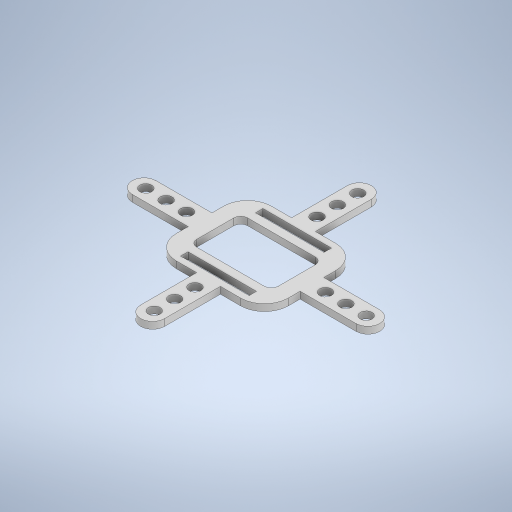
# Autodesk Inventor part: SoporteMarkers12
Saved by Autodesk Inventor 2024.3 (Build 283343000, 343)
## iProperties
Created: 2024-07-19
Part Number: SoporteMarkers12
Material: Generic
Document SubType Name: Modeling
Designer: pjcaa
Density: 1 g/cm^3
Appearance: Default
Mass: 1.30972 g
Surface Area: 17.5643 cm^2
Volume: 1.30972 cm^3
Author: pjcaa
Autodesk Inventor part; units mm, degrees
ref_plane "YZ Plane" through (0, 0, 0) normal (1, 0, 0) x (0, 1, 0)
ref_plane "XZ Plane" through (0, 0, 0) normal (0, 1, 0) x (-1, 0, 0)
ref_plane "XY Plane" through (0, 0, 0) normal (0, 0, 1) x (1, 0, 0)
sketch "Sketch1" plane through (0, 0, 0) normal (0, 1, 0) x (-1, 0, 0)
  line L0 (0, 0) -> (33, 0)
  line L1 (33, 0) -> (33, -28)
  line L2 (33, -28) -> (0, -28)
  line L3 (0, -28) -> (0, 0)
  line L4 (0, -17.5) -> (-20, -17.5)
  line L5 (-20, -17.5) -> (-20, -10.5)
  line L6 (-20, -10.5) -> (0, -10.5)
  line L7 (0, -10.5) -> (0, -17.5)
  line L8 (33, -17.5) -> (53, -17.5)
  line L9 (53, -17.5) -> (53, -10.5)
  line L10 (53, -10.5) -> (33, -10.5)
  line L11 (33, -10.5) -> (33, -17.5)
  line L12 (20, -28) -> (13, -28)
  line L13 (13, -28) -> (13, -48)
  line L14 (13, -48) -> (20, -48)
  line L15 (20, -48) -> (20, -28)
  line L16 (20, 0) -> (13, 0)
  line L17 (13, 0) -> (13, 20)
  line L18 (13, 20) -> (20, 20)
  line L19 (20, 20) -> (20, 0)
  circle A0 centre (16.5, -44) radius 1.75
  circle A1 centre (-16, -14) radius 1.75
  circle A2 centre (16.5, 16) radius 1.75
  circle A3 centre (49, -14) radius 1.75
  line L20 (16.5, -44) -> (16.5, -48) construction
  line L21 (-16, -14) -> (-20, -14) construction
  line L22 (16.5, 16) -> (16.5, 20) construction
  line L23 (49, -14) -> (53, -14) construction
  circle A4 centre (43, -14) radius 1.75
  circle A5 centre (37, -14) radius 1.75
  circle A6 centre (16.5, -38) radius 1.75
  circle A7 centre (16.5, -32) radius 1.75
  circle A8 centre (-10, -14) radius 1.75
  circle A9 centre (-4, -14) radius 1.75
  circle A10 centre (16.5, 10) radius 1.75
  circle A11 centre (16.5, 4) radius 1.75
  point P0 (16.5, -28)
  point P1 (16.5, 0)
  point P2 (0, -14)
  point P3 (33, -14)
  dimension "d0" = 33
  dimension "d1" = 28
  dimension "d29" = 7
  dimension "d34" = 20
  dimension "d35" = 4
  dimension "d36" = 3.5
  dimension "d44" = 6
  dimension "d51" = 6
  dimension "d58" = 6
  dimension "d65" = 6
  constraints: 48 end point, 14 perpendicular, 12 centre point, 12 midpoint, 10 parallel, 7 horizontal, 3 equal radius, 3 vertical alignment, 2 horizontal alignment, 2 vertical, 16 other
  measures "d0" distance of L1.end L2.end
  measures "d1" distance of L0.end L1.end
  measures "d29" distance of L8.end L9.end
  measures "d34" distance of L9.end L10.end
  measures "d35" distance of L20.start L20.end
  measures "d36" diameter of A0
  measures "d44" distance of L23.start A4.centre
  measures "d51" distance of L20.start A6.centre
  measures "d58" distance of L21.start A8.centre
  measures "d65" distance of L22.start A10.centre
extrude "Extrusion1" add sketch "Sketch1" along normal blind 2
sketch "Sketch2" plane through (0, 2, 0) normal (0, 1, 0) x (1, 0, 0)
  line L0 (0, 28) -> (-13, 28) projected
  line L1 (-33, 28) -> (-33, 17.5) projected
  line L2 (-33, 0) -> (-20, 0) projected
  line L3 (0, 0) -> (0, 10.5) projected
  line L4 (-26.6, 1.85) -> (-6.4, 1.85)
  line L5 (-6.4, 1.85) -> (-6.4, 4.05)
  line L6 (-6.4, 4.05) -> (-26.6, 4.05)
  line L7 (-26.6, 4.05) -> (-26.6, 1.85)
  line L8 (-26.6, 23.95) -> (-6.4, 23.95)
  line L9 (-6.4, 23.95) -> (-6.4, 26.15)
  line L10 (-6.4, 26.15) -> (-26.6, 26.15)
  line L11 (-26.6, 26.15) -> (-26.6, 23.95)
  line L12 (-26.6, 1.85) -> (-33, 1.85)
  line L13 (-26.6, 1.85) -> (-26.6, 0)
  line L14 (-26.6, 26.15) -> (-26.6, 28)
  line L15 (-6.4, 4.05) -> (0, 4.05)
  line L16 (-13, 28) -> (-13, 48) projected
  line L17 (-13, 48) -> (-20, 48) projected
  line L18 (-20, 48) -> (-20, 28) projected
  line L19 (-20, 28) -> (-33, 28) projected
  line L20 (-33, 17.5) -> (-53, 17.5) projected
  line L21 (-53, 17.5) -> (-53, 10.5) projected
  line L22 (-53, 10.5) -> (-33, 10.5) projected
  line L23 (-33, 10.5) -> (-33, 0) projected
  line L24 (-20, 0) -> (-20, -20) projected
  line L25 (-20, -20) -> (-13, -20) projected
  line L26 (-13, -20) -> (-13, 0) projected
  line L27 (-13, 0) -> (0, 0) projected
  line L28 (0, 10.5) -> (20, 10.5) projected
  line L29 (20, 10.5) -> (20, 17.5) projected
  line L30 (20, 17.5) -> (0, 17.5) projected
  line L31 (0, 17.5) -> (0, 28) projected
  line L32 (-28.5, 21.5) -> (-4.5, 21.5)
  line L33 (-4.5, 21.5) -> (-4.5, 6.5)
  line L34 (-4.5, 6.5) -> (-28.5, 6.5)
  line L35 (-28.5, 6.5) -> (-28.5, 21.5)
  line L36 (-28.5, 21.5) -> (-4.5, 6.5) construction
  line L37 (-4.5, 21.5) -> (-28.5, 6.5) construction
  point P0 (-16.5, 14)
  point P1 (-16.5, 23.95)
  point P2 (20, 14)
  dimension "d4" = 2.2
  dimension "d5" = 20.2
  dimension "d6" = 19.9
  dimension "d37" = 24
  dimension "d38" = 15
  constraints: 36 end point, 6 parallel, 5 perpendicular, 5 point on line, 4 equal length, 4 midpoint, 3 horizontal, 2 vertical alignment, 1 horizontal alignment, 1 vertical
  measures "d4" distance of L6.end L4.start
  measures "d5" distance of L4.start L4.end
  measures "d6" distance between parallel lines of L8 L6
  measures "d37" distance of L33.end L34.end
  measures "d38" distance of L32.end L33.end
extrude "Extrusion2" cut sketch "Sketch2" against normal through all contours L10 L9 L8 L11 | L5 L4 L7 L6 | L32 L33 L34 L35
fillet "Fillet1" radius 3.5 8 edges at (-20, 1, 20) (-13, 1, 20) (20, 1, -10.5) (20, 1, -17.5) (-13, 1, -48) (-20, 1, -48) (-53, 1, -17.5) (-53, 1, -10.5)
fillet "Fillet2" radius 7 4 edges at (-33, 1, 0) (-33, 1, -28) (0, 1, -28) (0, 1, 0)
fillet "Fillet3" radius 2 4 edges at (-28.5, 1, -21.5) (-4.5, 1, -21.5) (-28.5, 1, -6.5) (-4.5, 1, -6.5)
sketch "Sketch4" plane through (0, 2, 0) normal (0, 1, 0) x (1, 0, 0)
  arc A0 (-4.5, 19.5) -> (-6.5, 21.5) centre (-6.5, 19.5) ccw construction
  line L0 (-26.5, 21.5) -> (-6.5, 21.5) construction
  line L1 (-4.5, 19.5) -> (-4.5, 8.5) construction
  arc A1 (-6.5, 6.5) -> (-4.5, 8.5) centre (-6.5, 8.5) ccw construction
  line L2 (-6.5, 6.5) -> (-26.5, 6.5) construction
  arc A2 (-28.5, 8.5) -> (-26.5, 6.5) centre (-26.5, 8.5) ccw construction
  line L3 (-28.5, 8.5) -> (-28.5, 19.5) construction
  arc A3 (-26.5, 21.5) -> (-28.5, 19.5) centre (-26.5, 19.5) ccw construction
  line L4 (-25.5, 21.5) -> (-23.5, 21.5)
  line L5 (-23.5, 21.5) -> (-23.5, 6.5)
  line L6 (-23.5, 6.5) -> (-25.5, 6.5)
  line L7 (-25.5, 6.5) -> (-25.5, 21.5)
  line L8 (-9.5, 6.5) -> (-7.5, 6.5)
  line L9 (-7.5, 6.5) -> (-7.5, 21.5)
  line L10 (-7.5, 21.5) -> (-9.5, 21.5)
  line L11 (-9.5, 21.5) -> (-9.5, 6.5)
  point P0 (0, 0)
  dimension "d70" = 3
  dimension "d71" = 3
  dimension "d72" = 2
  constraints: 16 end point, 4 parallel, 4 point on line, 2 horizontal, 2 perpendicular, 1 collinear
  measures "d70" distance between parallel lines of L3 L7
  measures "d71" distance between parallel lines of L1 L9
  measures "d72" distance between parallel lines of L7 L5
body "Solid1"
